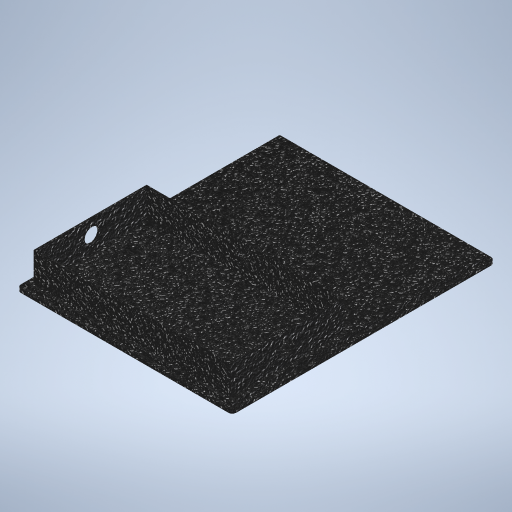
# Autodesk Inventor part: tapa caja arduino
Saved by Autodesk Inventor 2023 (Build 270158000, 158)
## iProperties
Created: 2022-10-27
Part Number: tapa caja arduino
Material: Generic
Document SubType Name: Modeling
Designer: Xiaba
Density: 1 g/cm^3
Appearance: Default
Author: Xiaba
Autodesk Inventor part; units mm, degrees
ref_plane "YZ Plane" through (0, 0, 0) normal (1, 0, 0) x (0, 1, 0)
ref_plane "XZ Plane" through (0, 0, 0) normal (0, 1, 0) x (-1, 0, 0)
ref_plane "XY Plane" through (0, 0, 0) normal (0, 0, 1) x (1, 0, 0)
sketch "Sketch1" plane through (0, 0, 0) normal (0, 1, 0) x (-1, 0, 0)
  line L0 (1, 0) -> (58, 0)
  line L1 (59, -1) -> (59, -71)
  line L2 (58, -72) -> (1, -72)
  line L3 (0, -71) -> (0, -1)
  arc A0 (59, -1) -> (58, 0) centre (58, -1) ccw
  arc A1 (58, -72) -> (59, -71) centre (58, -71) ccw
  arc A2 (0, -71) -> (1, -72) centre (1, -71) ccw
  arc A3 (1, 0) -> (0, -1) centre (1, -1) ccw
  point P0 (0, 0)
  point P1 (59, -72)
  point P2 (59, 0)
  point P3 (0, -72)
  dimension "d0" = 72
  dimension "d1" = 59
  dimension "d2" = 1
  constraints: 8 end point, 8 point on circle, 8 point on line, 8 tangent, 4 centre point, 3 equal radius, 2 parallel, 1 horizontal, 1 perpendicular
  measures "d0" distance of point (59, 0) point (59, -72)
  measures "d1" distance of point (59, -72) point (0, -72)
  measures "d2" radius of A0
extrude "Extrusion1" add sketch "Sketch1" along normal blind 1
sketch "Sketch2" plane through (0, 1, 0) normal (0, 1, 0) x (1, 0, 0)
  line L0 (-55.9113, 2.4272) -> (-2.9113, 2.4272)
  line L1 (-2.9113, 2.4272) -> (-2.9113, 32.4272)
  line L2 (-2.9113, 32.4272) -> (-55.9113, 32.4272)
  line L3 (-55.9113, 32.4272) -> (-55.9113, 2.4272)
  line L4 (-56.4113, 1.9272) -> (-2.4113, 1.9272)
  line L5 (-2.4113, 1.9272) -> (-2.4113, 32.9272)
  line L6 (-2.4113, 32.9272) -> (-56.4113, 32.9272)
  line L7 (-56.4113, 32.9272) -> (-56.4113, 1.9272)
  point P0 (0, 0)
  dimension "d5" = 30
  dimension "d6" = 53
  dimension "d7" = 0.5
  dimension "d8" = 0.5
  dimension "d9" = 0.5
  dimension "d10" = 0.5
  constraints: 16 end point, 4 parallel, 2 horizontal, 2 perpendicular
  measures "d5" distance of L2.end L0.start
  measures "d6" distance of L0.start L0.end
  measures "d7" distance between parallel lines of L6 L2
  measures "d8" distance between parallel lines of L3 L7
  measures "d9" distance between parallel lines of L4 L0
  measures "d10" distance between parallel lines of L5 L1
extrude "Extrusion2" add sketch "Sketch2" along normal blind 4
sketch "Sketch3" plane through (0, 1, 0) normal (0, 1, 0) x (1, 0, 0)
  arc A0 (0, 71) -> (-1, 72) centre (-1, 71) ccw projected
  line L0 (-58, 1) -> (-1, 1)
  line L1 (-1, 1) -> (-1, 71)
  line L2 (-1, 71) -> (-58, 71)
  line L3 (-58, 71) -> (-58, 1)
  line L4 (-1, 72) -> (-58, 72) projected
  line L5 (-59, 71) -> (-59, 1) projected
  line L6 (-58, 0) -> (-1, 0) projected
  line L7 (0, 1) -> (0, 71) projected
  point P0 (0, 0)
  dimension "d13" = 1
  dimension "d14" = 1
  dimension "d15" = 1
  dimension "d16" = 1
  constraints: 8 end point, 2 parallel, 1 horizontal, 1 perpendicular
  measures "d13" distance between parallel lines of L4 L2
  measures "d14" distance between parallel lines of L5 L3
  measures "d15" distance between parallel lines of L6 L0
  measures "d16" distance between parallel lines of L7 L1
extrude "Extrusion3" add sketch "Sketch3" along normal blind 1
sketch "Sketch4" plane through (0, 5, 0) normal (0, 1, 0) x (1, 0, 0)
  line L0 (-2.4113, 1.9272) -> (-2.4113, 32.9272) projected
  line L1 (-2.9113, 32.4272) -> (-2.9113, 2.4272) projected
  line L2 (-56.4113, 1.9272) -> (-2.4113, 1.9272) projected
  line L3 (-2.9113, 2.4272) -> (-55.9113, 2.4272) projected
  line L4 (-2.4113, 32.9272) -> (-56.4113, 32.9272) projected
  line L5 (-55.9113, 32.4272) -> (-2.9113, 32.4272) projected
  line L6 (-55.9113, 2.4272) -> (-55.9113, 32.4272) projected
  line L7 (-56.4113, 32.9272) -> (-56.4113, 1.9272) projected
  point P0 (0, 0)
extrude "Extrusion4" add sketch "Sketch4" along normal blind 5
sketch "Sketch5" plane through (-2.4113, 2, -1.9272) normal (1, 0, 0) x (0, 0, -1)
  line L0 (0, 0) -> (31, 0) projected
  line L1 (31, 0) -> (31, 8) projected
  line L2 (0, 8) -> (31, 8) projected
  line L3 (0, 0) -> (0, 8) projected
  circle A0 centre (15.5, 4) radius 2
  point P0 (-1.9272, -2)
  dimension "d21" = 4
  constraints: 1 centre point
  measures "d21" diameter of A0
extrude "Extrusion6" cut sketch "Sketch5" against normal through all contours A0
sketch "Sketch7" plane through (-2.4113, 2, -32.9272) normal (0, 0, -1) x (-1, 0, 0)
  line L0 (0, 0) -> (54, 0) projected
  line L1 (54, 0) -> (54, 8) projected
  line L2 (0, 8) -> (54, 8) projected
  line L3 (0, 0) -> (0, 8) projected
  circle A0 centre (27, 4) radius 1.5
  point P0 (-2.4113, -2)
  dimension "d26" = 3
  constraints: 1 centre point
  measures "d26" diameter of A0
extrude "Extrusion7" cut sketch "Sketch7" against normal blind 3 contours A0
body "Solid1"
